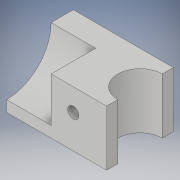
# Autodesk Inventor part: Part4
Saved by Autodesk Inventor 2017 (Build 210142000, 142)
## iProperties
Created: 2016-11-03
Part Number: Part4
Material: Generic
Document SubType Name: Modeling
Designer: s411888
Density: 1 g/cm^3
Appearance: Default
Author: s411888
Autodesk Inventor part; units mm, degrees
ref_plane "YZ Plane" through (0, 0, 0) normal (1, 0, 0) x (0, 1, 0)
ref_plane "XZ Plane" through (0, 0, 0) normal (0, 1, 0) x (-1, 0, 0)
ref_plane "XY Plane" through (0, 0, 0) normal (0, 0, 1) x (1, 0, 0)
sketch "Sketch1" plane through (0, 0, 0) normal (0, 1, 0) x (-1, 0, 0)
  line L0 (36.9116, 5.5131) -> (-20.2384, 5.5131)
  line L1 (-20.2384, 5.5131) -> (-20.2384, -32.5869)
  line L2 (-20.2384, -32.5869) -> (36.9116, -32.5869)
  line L3 (36.9116, -32.5869) -> (36.9116, 5.5131)
  point P0 (0, 0)
  dimension "d0" = 57.15
  dimension "d1" = 38.1
  constraints: 8 end point, 2 parallel, 1 horizontal, 1 perpendicular
  measures "d0" distance of L2.end L1.end
  measures "d1" distance of L1.end L0.end
extrude "Extrusion1" add sketch "Sketch1" along normal blind 31.75
sketch "Sketch2" plane through (0, 31.75, 0) normal (0, 1, 0) x (1, 0, 0)
  line L0 (-36.9116, -5.5131) -> (20.2384, -5.5131) projected
  line L1 (20.2384, -5.5131) -> (1.1884, -5.5131)
  line L2 (1.1884, -5.5131) -> (1.1884, 13.5369)
  line L3 (1.1884, 13.5369) -> (20.2384, 13.5369)
  line L4 (20.2384, 13.5369) -> (20.2384, -5.5131)
  line L5 (20.2384, -5.5131) -> (20.2384, 32.5869) projected
  line L6 (20.2384, 32.5869) -> (1.1884, 32.5869)
  line L7 (1.1884, 32.5869) -> (1.1884, 13.5369)
  line L8 (1.1884, 13.5369) -> (20.2384, 13.5369)
  line L9 (20.2384, 13.5369) -> (20.2384, 32.5869)
  point P0 (0, 0)
  dimension "d4" = 19.05
  dimension "d5" = 19.05
  dimension "d6" = 19.05
  dimension "d7" = 19.05
  constraints: 16 end point, 4 parallel, 2 horizontal, 2 perpendicular
  measures "d4" distance of L2.end L3.end
  measures "d5" distance of L1.end L2.end
  measures "d6" distance of L8.end L7.end
  measures "d7" distance of L7.end L6.end
sketch "Sketch3" plane through (0, 31.75, 0) normal (0, 1, 0) x (1, 0, 0)
  line L0 (20.2384, -5.5131) -> (20.2384, 32.5869) projected
  circle A0 centre (20.2384, 13.5369) radius 12.7
  point P0 (0, 0)
  dimension "d8" = 25.4
  constraints: 1 centre point, 1 midpoint
  measures "d8" diameter of A0
extrude "Extrusion2" cut sketch "Sketch3" against normal blind 31.75
sketch "Sketch5" plane through (-36.9116, 0, -32.5869) normal (-1, 0, 0) x (0, 0, 1)
  line L0 (0, 0) -> (38.1, 0) projected
  line L1 (38.1, 0) -> (31.75, 0)
  line L2 (31.75, 0) -> (31.75, 6.35)
  line L3 (31.75, 6.35) -> (38.1, 6.35)
  line L4 (38.1, 6.35) -> (38.1, 0)
  line L5 (38.1, 0) -> (38.1, 31.75) projected
  circle A0 centre (38.1, 31.75) radius 25.4
  point P0 (32.5869, 0)
  dimension "d13" = 6.35
  dimension "d14" = 6.35
  dimension "d15" = 50.8
  constraints: 8 end point, 2 parallel, 1 centre point, 1 horizontal, 1 perpendicular
  measures "d13" distance of L2.end L3.end
  measures "d14" distance of L1.end L2.end
  measures "d15" diameter of A0
extrude "Extrusion3" cut sketch "Sketch5" against normal blind 25.4 contours A0
sketch "Sketch6" plane through (-36.9116, 0, 5.5131) normal (0, 0, 1) x (1, 0, 0)
  line L0 (25.4, 31.75) -> (57.15, 31.75) projected
  circle A0 centre (38.1, 19.05) radius 3.175
  point P0 (36.9116, 0)
  dimension "d20" = 6.35
  constraints: 1 centre point
  measures "d20" diameter of A0
extrude "Extrusion4" cut sketch "Sketch6" against normal blind 50.8
body "Solid1"
